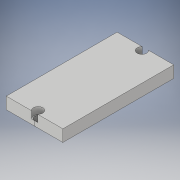
# Autodesk Inventor part: Bottom
Saved by Autodesk Inventor 2019 (Build 230136000, 136)
## iProperties
Created: 2020-02-01
Part Number: Bottom
Material: Generic
Document SubType Name: Modeling
Designer: alb16148
Density: 1 g/cm^3
Appearance: Default
Author: alb16148
Autodesk Inventor part; units mm, degrees
ref_plane "YZ Plane" through (0, 0, 0) normal (1, 0, 0) x (0, 1, 0)
ref_plane "XZ Plane" through (0, 0, 0) normal (0, 1, 0) x (-1, 0, 0)
ref_plane "XY Plane" through (0, 0, 0) normal (0, 0, 1) x (1, 0, 0)
sketch "Sketch1" plane through (0, 0, 0) normal (0, 1, 0) x (-1, 0, 0)
  line L0 (12, 23.5) -> (-12, 23.5)
  line L1 (-12, 23.5) -> (-12, -23.5)
  line L2 (-12, -23.5) -> (12, -23.5)
  line L3 (12, -23.5) -> (12, 23.5)
  point P0 (0, 0)
  dimension "d0" = 12
  dimension "d1" = 12
  dimension "d2" = 23.5
  dimension "d3" = 23.5
  constraints: 8 end point, 2 parallel, 1 horizontal, 1 perpendicular
  measures "d0" distance from line of L3 point (0, 0)
  measures "d1" distance from line of L1 point (0, 0)
  measures "d2" distance from line of L0 point (0, 0)
  measures "d3" distance from line of L2 point (0, 0)
extrude "Extrusion1" add sketch "Sketch1" along normal blind 5
sketch "Sketch2" plane through (0, 5, 0) normal (0, 1, 0) x (1, 0, 0)
  circle A0 centre (0, -22) radius 1.5
  circle A1 centre (0, 22) radius 1.5
  point P0 (0, 0)
  dimension "d6" = 3
  dimension "d7" = 3
  dimension "d8" = 22
  dimension "d9" = 22
  dimension "d10" = 0
  dimension "d11" = 0
  constraints: 2 centre point
  measures "d6" diameter of A0
  measures "d7" diameter of A1
  measures "d8" distance of A0.centre point (0, 0)
  measures "d9" distance of point (0, 0) A1.centre
  measures "d10" horizontal distance of point (0, 0) A0.centre
  measures "d11" horizontal distance of point (0, 0) A1.centre
extrude "Extrusion2" cut sketch "Sketch2" against normal up to surface (5 mm away)
sketch "Sketch4" plane through (0, 5, 0) normal (0, 1, 0) x (1, 0, 0)
  circle A0 centre (0, -22) radius 1.5 projected
  circle A1 centre (0, 22) radius 1.5 projected
  line L0 (-12, -23.5) -> (0, -23.5) projected
  line L1 (12, -23.5) -> (12, 23.5) projected
  line L2 (12, 23.5) -> (0, 23.5) projected
  line L3 (-12, 23.5) -> (-12, -23.5) projected
  circle A2 centre (0, -22) radius 2
  circle A3 centre (0, 22) radius 2
  line L4 (0, -23.5) -> (12, -23.5) projected
  line L5 (0, 23.5) -> (-12, 23.5) projected
  point P0 (0, 0)
  dimension "d14" = 4
  dimension "d15" = 4
  constraints: 2 centre point, 2 coincident, 2 vertical alignment
  measures "d14" diameter of A2
  measures "d15" diameter of A3
extrude "Extrusion3" cut sketch "Sketch4" against normal blind 3 contours L0 A2 L4 | L4 A2 L0 | L5 L2 A3 | A3 L2 L5
sketch "Sketch5" plane through (0, 0, 0) normal (0, -1, 0) x (1, 0, 0)
  line L0 (6.9, -7.1144) -> (6.9, 7.2186) projected
  line L1 (6.9, 7.2186) -> (-8.137, 7.2) projected
  line L2 (-8.137, 7.2) -> (-8.104, -7.136) projected
  line L3 (-8.104, -7.136) -> (6.9, -7.1144) projected
  circle A0 centre (4.9456, 5.262) radius 0.4065 projected
  circle A1 centre (4.9282, -4.9331) radius 0.4065 projected
  circle A2 centre (4.9478, 2.722) radius 0.4065 projected
  circle A3 centre (4.952, -2.358) radius 0.4065 projected
  circle A4 centre (-6.0981, 4.9907) radius 1.5 projected
  circle A5 centre (-6.0897, -5.0423) radius 1.5 projected
  circle A6 centre (-6.0897, -5.0423) radius 1
  circle A7 centre (-6.0981, 4.9907) radius 1
  point P0 (0, 0)
  dimension "d24" = 1
  dimension "d25" = 1
  constraints: 2 centre point, 2 coincident
  measures "d24" radius of A6
  measures "d25" radius of A7
extrude "Extrusion4" add sketch "Sketch5" along normal blind 0.01 contours A4 | A5 | A6 | A7
sketch "Sketch6" plane through (0, 0, 0) normal (0, -1, 0) x (1, 0, 0)
  circle A0 centre (-6.0981, 4.9907) radius 1.5 projected
  circle A1 centre (-6.0897, -5.0423) radius 1.5 projected
  circle A2 centre (0, 22) radius 1.5 projected
  circle A3 centre (0, -22) radius 1.5 projected
  line L0 (-12, 23.5) -> (0, 23.5) projected
  line L1 (-12, -23.5) -> (-12, 23.5) projected
  line L2 (12, -23.5) -> (0, -23.5) projected
  line L3 (12, 23.5) -> (12, -23.5) projected
  circle A4 centre (-6.0981, 4.9907) radius 2.5
  circle A5 centre (-6.0897, -5.0423) radius 2.5
  line L4 (0, -23.5) -> (-12, -23.5) projected
  line L5 (0, 23.5) -> (12, 23.5) projected
  point P0 (0, 0)
  dimension "d20" = 1
  dimension "d21" = 1
  constraints: 2 centre point, 2 vertical alignment
  measures "d20" radial gap between concentric circles of A0 A4
  measures "d21" radial gap between concentric circles of A1 A5
extrude "Extrusion5" add sketch "Sketch6" along normal blind 2 contours A4 | A5
sketch "Sketch7" plane through (-6.0897, -2, -5.0423) normal (0, -1, 0) x (1, 0, 0)
  circle A0 centre (0, 0) radius 1.5 projected
  circle A1 centre (0, 0) radius 2.5 projected
  circle A2 centre (-0.0084, 10.033) radius 1.5 projected
  circle A3 centre (-0.0084, 10.033) radius 2.5 projected
  circle A4 centre (0, 0) radius 1
  circle A5 centre (-0.0084, 10.033) radius 1
  point P0 (6.0897, 5.0423)
  dimension "d26" = 1
  dimension "d27" = 1
  constraints: 2 centre point, 2 coincident
  measures "d26" radius of A4
  measures "d27" radius of A5
extrude "Extrusion6" add sketch "Sketch7" against normal blind 5 contours A0 | A2
equation "\"d1\" = d0"
body "Solid1"
